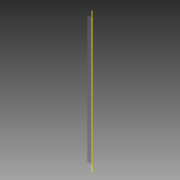
# Autodesk Inventor part: GuardShield
Saved by Autodesk Inventor 2013 (Build 170138000, 138)
## iProperties
Created: 2013-01-07
Part Number: GuardShield
Material: Polycarbonate, Clear
Document SubType Name: Modeling
Designer: Phillip
Density: 1 g/cm^3
Author: Phillip
Autodesk Inventor part; units mm, degrees
ref_plane "YZ Plane" through (0, 0, 0) normal (1, 0, 0) x (0, 1, 0)
ref_plane "XZ Plane" through (0, 0, 0) normal (0, 1, 0) x (-1, 0, 0)
ref_plane "XY Plane" through (0, 0, 0) normal (0, 0, 1) x (1, 0, 0)
ref_plane "Work Plane1" through (0, 0, 0) normal (0, 0, 1) x (1, 0, 0)
sketch "Sketch1" plane through (0, 0, 0) normal (0, 0, 1) x (1, 0, 0)
  line L0 (0, 0) -> (0, 13016.611) projected
  line L1 (0, 0) -> (-541.401, 0)
  line L2 (-541.401, 0) -> (-541.401, 13050.012)
  line L3 (-541.401, 13050.012) -> (0, 13050.012)
  line L4 (0, 0) -> (-541.401, 0)
  line L5 (-541.401, 0) -> (-541.401, 13050.012)
  line L6 (-541.401, 13050.012) -> (0, 13050.012)
  line L7 (0, 13050.012) -> (0, 0)
  constraints: 14 end point, 3 horizontal, 2 parallel, 1 perpendicular, 1 vertical, 5 other
extrude "Extrusion1" add sketch "Sketch1" along normal blind 6.35
body "Solid1"
